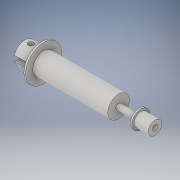
# Autodesk Inventor part: shaft
Saved by Autodesk Inventor 2017 (Build 210142000, 142)
## iProperties
Created: 2017-01-30
Part Number: shaft
Material: Generic
Document SubType Name: Modeling
Designer: yul067
Density: 1 g/cm^3
Appearance: Default
Author: yul067
Autodesk Inventor part; units mm, degrees
ref_plane "YZ Plane" through (0, 0, 0) normal (1, 0, 0) x (0, 1, 0)
ref_plane "XZ Plane" through (0, 0, 0) normal (0, 1, 0) x (-1, 0, 0)
ref_plane "XY Plane" through (0, 0, 0) normal (0, 0, 1) x (1, 0, 0)
sketch "Sketch1" plane through (0, 0, 0) normal (1, 0, 0) x (0, 1, 0)
  circle A0 centre (0, 0) radius 6
  dimension "d0" = 12
  constraints: 1 centre point, 1 coincident
  measures "d0" diameter of A0
extrude "Extrusion1" add sketch "Sketch1" along normal blind 52.5
sketch "Sketch2" plane through (52.5, 0, 0) normal (1, 0, 0) x (0, 0, -1)
  circle A0 centre (0, 0) radius 1.5
  dimension "d3" = 3
  constraints: 1 centre point, 1 coincident
  measures "d3" diameter of A0
extrude "Extrusion2" add sketch "Sketch2" along normal blind 11.5
sketch "Sketch3" plane through (64, 0, 0) normal (1, 0, 0) x (0, 0, -1)
  circle A0 centre (0, 0) radius 5
  dimension "d6" = 10
  constraints: 1 centre point, 1 coincident
  measures "d6" diameter of A0
extrude "Extrusion3" add sketch "Sketch3" along normal blind 1
sketch "Sketch4" plane through (65, 0, 0) normal (1, 0, 0) x (0, 0, -1)
  circle A0 centre (0, 0) radius 3.75
  dimension "d9" = 7.5
  constraints: 1 centre point, 1 coincident
  measures "d9" diameter of A0
extrude "Extrusion4" add sketch "Sketch4" along normal blind 8
sketch "Sketch5" plane through (73, 0, 0) normal (1, 0, 0) x (0, 0, -1)
  circle A0 centre (0, 0) radius 1.5
  dimension "d12" = 3
  constraints: 1 centre point, 1 coincident
  measures "d12" diameter of A0
extrude "Extrusion5" cut sketch "Sketch5" against normal blind 8
sketch "Sketch6" plane through (0, 0, 0) normal (-1, 0, 0) x (0, 0, 1)
  circle A0 centre (0, 0) radius 3.75 projected
  circle A1 centre (0, 0) radius 5.5
  circle A2 centre (0, 0) radius 1.5 projected
  circle A3 centre (0, 0) radius 6
  dimension "d15" = 11
  dimension "d16" = 12
  constraints: 2 centre point, 2 coincident
  measures "d15" diameter of A1
  measures "d16" diameter of A3
extrude "Extrusion6" cut sketch "Sketch6" against normal blind 10.5 contours A3
sketch "Sketch7" plane through (10.5, 0, 0) normal (-1, 0, 0) x (0, 0, 1)
  circle A0 centre (0, 0) radius 10
  dimension "d19" = 20
  constraints: 1 centre point, 1 coincident
  measures "d19" diameter of A0
extrude "Extrusion7" add sketch "Sketch7" along normal blind 1
sketch "Sketch8" plane through (0, 0, 0) normal (-1, 0, 0) x (0, 0, 1)
  line L0 (-6, 1.5) -> (6, 1.5)
  line L1 (6, 1.5) -> (6, -1.5)
  line L2 (6, -1.5) -> (-6, -1.5)
  line L3 (-6, -1.5) -> (-6, 1.5)
  line L4 (-6, 1.5) -> (6, -1.5) construction
  line L5 (6, 1.5) -> (-6, -1.5) construction
  point P0 (0, 0)
  point P1 (0, 0)
  dimension "d23" = 12
  constraints: 12 end point, 2 midpoint, 2 parallel, 1 horizontal, 1 perpendicular
  measures "d23" distance of L1.end L2.end
extrude "Extrusion8" cut sketch "Sketch8" against normal blind 9
sketch "Sketch10" plane through (9.5, 0, 0) normal (-1, 0, 0) x (0, 0, 1)
  circle A0 centre (0, 0) radius 6
  circle A1 centre (0, 0) radius 1.5 projected
  circle A2 centre (0, 0) radius 4.8442
  constraints: 2 centre point, 2 coincident
extrude "Extrusion10" add sketch "Sketch10" along normal blind 9.5 contours A0
sketch "Sketch12" plane through (0, 0, 0) normal (-1, 0, 0) x (0, 0, 1)
  line L0 (-8.4132, -1.5) -> (8.4132, -1.5)
  line L1 (8.4132, -1.5) -> (8.4132, 1.5)
  line L2 (8.4132, 1.5) -> (-8.4132, 1.5)
  line L3 (-8.4132, 1.5) -> (-8.4132, -1.5)
  line L4 (-8.4132, -1.5) -> (8.4132, 1.5) construction
  line L5 (8.4132, -1.5) -> (-8.4132, 1.5) construction
  point P0 (0, 0)
  dimension "d35" = 3
  constraints: 12 end point, 2 midpoint, 2 parallel, 1 horizontal, 1 perpendicular
  measures "d35" distance of L1.end L0.end
extrude "Extrusion12" cut sketch "Sketch12" against normal blind 9
sketch "Sketch13" plane through (0, 1.5, -5.8095) normal (0, -1, 0) x (1, 0, 0)
  line L0 (-3.5, 6.3202) -> (3.5, 6.3202)
  line L1 (3.5, 6.3202) -> (3.5, 5.2988)
  line L2 (3.5, 5.2988) -> (-3.5, 5.2988)
  line L3 (-3.5, 5.2988) -> (-3.5, 6.3202)
  line L4 (-3.5, 6.3202) -> (3.5, 5.2988) construction
  line L5 (3.5, 6.3202) -> (-3.5, 5.2988) construction
  circle A0 centre (3.5, 5.8095) radius 1.5
  point P0 (0, 5.8095)
  dimension "d38" = 7
  dimension "d39" = 3
  constraints: 12 end point, 3 midpoint, 2 parallel, 1 centre point, 1 horizontal, 1 perpendicular
  measures "d38" distance of L1.end L2.end
  measures "d39" diameter of A0
extrude "Extrusion13" cut sketch "Sketch13" along normal through all both and the other way through all contours A0 L2 L1 L0 | L0 L1 L2 A0
body "Solid1"
